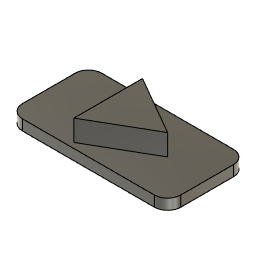
yieldSignPiece (Autodesk Fusion 360 archive; units mm, degrees)
design "yieldSign" references "TactileMapsParameters"
Autodesk Fusion 360 part; units mm, degrees
derive "ExternalDerived1" from "TactileMapsParameters v5"
sketch "Sketch1" plane through (0, 0, 0) normal (0, 0, 1) x (1, 0, 0)
  line L0 (0, 0) -> (12, 0)
  line L1 (12, 0) -> (12, 6)
  line L2 (12, 6) -> (0, 6)
  line L3 (0, 6) -> (0, 0)
  dimension "d24" = 12
  dimension "d25" = 6
  constraint horizontal L0
  constraint vertical L1
  constraint horizontal L2
  constraint vertical L3
  constraint coincident L0.start L3.end
  measures "d24" distance of L0.start L0.end
  measures "d25" distance of L0.start L2.end
extrude "Extrude3" add sketch "Sketch1" along normal blind 0.8
sketch "Sketch3" plane through (0, 0, 0.8) normal (0, 0, 1) x (-1, 0, 0)
  line L0 (0, -6) -> (0, 0)
  line L1 (0, 0) -> (-12, 0)
  line L2 (-12, 0) -> (-12, -6)
  line L3 (-12, -6) -> (0, -6)
  line L4 (0, -3) -> (-12, -3) construction
  line L5 (-6, 0) -> (-6, -6) construction
  line L6 (-9, -3) -> (-4.5, -5.5981)
  line L7 (-4.5, -5.5981) -> (-4.5, -0.4019)
  line L8 (-4.5, -0.4019) -> (-9, -3)
  point P0 (-6, -3)
  dimension "d28" = 3
  constraint midpoint L0 L4.start
  constraint midpoint L2 L4.end
  constraint midpoint L1 L5.start
  constraint midpoint L3 L5.end
  constraint coincident L4 L6.start
  constraint midpoint L4 P0
  measures "d28" distance of L6.start P0
extrude "Extrude4" add sketch "Sketch3" along normal blind 1.6 contours L6 L7 L8
fillet "Fillet1" radius 1 4 edges at (0, 0, 0.4) (0, 6, 0.4) (12, 0, 0.4) (12, 6, 0.4)
equation "length_Ref = 170 mm" comment "Side lengths of base of model"
equation "baseHeight_Ref = 0.4 mm" comment "Height of the base of the model"
equation "sidewalkHeight_Ref = 3.2 mm" comment "Height of sidewalk/walking surface"
equation "sidewalkWidth_Ref = length_Ref / 3" comment "Width of the sidewalk/walking surface"
equation "orientorSize_Ref = 6 mm" comment "Side length of orientation indicator square"
equation "oritentorHeight_Ref = 2.4 mm" comment "Height of the orientation indicator"
equation "braileHeight_Ref = 0.6 mm" comment "Standard height of Braille characters"
equation "filletRadius_Ref = 0.6 mm" comment "Radius of fillets to soften edges"
equation "lineWidth_Ref = 3 mm" comment "Width of crosswalk lines"
equation "lineHeight_Ref = braileHeight_Ref / 2" comment "Height of crosswalk lines"
equation "tabWidth_Ref = length_Ref / 10" comment "Width of tabs to secure adjacent maps together"
equation "tabLength_Ref = length_Ref / 14" comment "Length of tab to secure adjacent maps together"
equation "tabHeight_Ref = sidewalkHeight_Ref / 4" comment "Height of tabs to secure adjacent maps together"
equation "clearance_Ref = 0.4 mm" comment "Clearance around parts that will fit together"
equation "featureHeight_Ref = 1.6 mm" comment "Height of features such as bus stops"
equation "pegSize_Ref = 6 mm" comment "Side length of pegs/holes to connect features to map base"
equation "pegDepth_Ref = sidewalkHeight_Ref / 4" comment "Depth of pegs/holes to connect features to map base"
equation "d24 = 2 * pegSize_Ref"
equation "d25 = pegSize_Ref"
equation "d26 = pegDepth_Ref"
equation "d28 = pegSize_Ref / 2"
equation "d29 = featureHeight_Ref"
